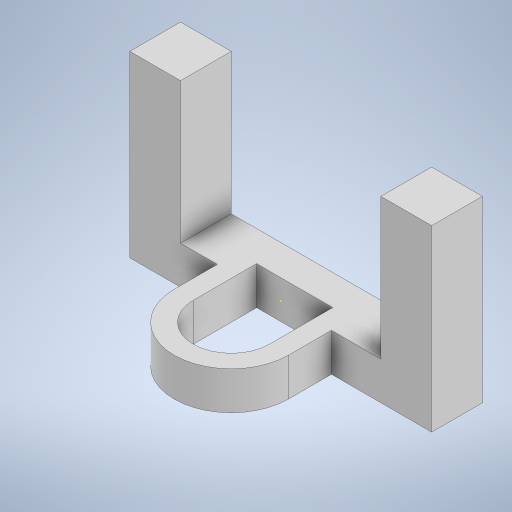
# Autodesk Inventor part: 액추에이터 지지대 3D 프린트
Saved by Autodesk Inventor 2024 (Build 280153000, 153)
## iProperties
Created: 2024-06-08
Part Number: 액추에이터 지지대 3D 프린트
Material: 일반
Document SubType Name: Modeling
Designer: kkamin5
Density: 1 g/cm^3
Appearance: 기본값
Author: kkamin5
Autodesk Inventor part; units mm, degrees
ref_plane "YZ Plane" through (0, 0, 0) normal (1, 0, 0) x (0, 1, 0)
ref_plane "XZ Plane" through (0, 0, 0) normal (0, 1, 0) x (-1, 0, 0)
ref_plane "XY Plane" through (0, 0, 0) normal (0, 0, 1) x (1, 0, 0)
sketch "스케치1" plane through (0, 0, 0) normal (0, 1, 0) x (-1, 0, 0)
  arc A0 (25, 17) -> (-20, 17) centre (2.5, 17) ccw
  arc A1 (17.5, 17) -> (-12.5, 17) centre (2.5, 17) ccw
  line L0 (17.5, 17) -> (-12.5, 17)
  line L1 (-20, 17) -> (-20, 0)
  line L2 (-20, -20) -> (25, -20)
  line L3 (25, 0) -> (25, 17)
  line L4 (-12.5, 17) -> (17.5, 17)
  line L5 (17.5, 17) -> (17.5, 0)
  line L6 (17.5, 0) -> (-12.5, 0)
  line L7 (-12.5, 0) -> (-12.5, 17)
  line L8 (59.5, -20) -> (-59.5, -20)
  line L9 (-59.5, -20) -> (-59.5, 0)
  line L10 (59.5, 0) -> (59.5, -20)
  line L11 (25, 0) -> (59.5, 0)
  line L12 (-59.5, 0) -> (-20, 0)
  line L13 (-12.5, 0) -> (17.5, 0)
  line L14 (17.5, 0) -> (-12.5, 0)
  line L15 (-12.5, 0) -> (-12.5, -8)
  line L16 (-12.5, -8) -> (17.5, -8)
  line L17 (17.5, -8) -> (17.5, 0)
  point P0 (0, 0)
  point P1 (0, 17)
  point P2 (-59.5, -10)
  dimension "d1" = 30
  dimension "d2" = 45
  dimension "d3" = 0
  dimension "d4" = 17
  dimension "d5" = 37
  dimension "d6" = 119
  dimension "d10" = 20
  dimension "d11" = 22.5
  dimension "d12" = 0
  dimension "d13" = 59.5
  dimension "d14" = 8
  dimension "d15" = 39.5
  constraints: 36 end point, 10 parallel, 4 horizontal, 4 perpendicular, 4 point on circle, 3 collinear, 3 tangent, 2 centre point, 2 point on line, 1 coincident, 1 midpoint
  measures "d1" diameter of A1
  measures "d2" distance of L2.start L2.end
  measures "d3" horizontal distance of point (0, 17) point (0, 0)
  measures "d4" distance of L0.start L5.end
  measures "d5" distance of L2.end L3.end
  measures "d6" distance of L8.start L8.end
  measures "d10" distance of L10.start L8.start
  measures "d11" radius of A0
  measures "d12" distance from line of point (0, 0) L6
  measures "d13" distance from line of point (0, 0) L10
  measures "d14" distance of L15.end L14.end
  measures "d15" distance between parallel lines of L9 L1
extrude "돌출1" add sketch "스케치1" along normal blind 15
sketch "스케치2" plane through (0, 15, 0) normal (0, 1, 0) x (1, 0, 0)
  point P0 (0, 0)
sketch "스케치3" plane through (0, 15, 0) normal (0, 1, 0) x (1, 0, 0)
  line L0 (-39.5, 0) -> (-59.5, 0)
  line L1 (-59.5, 0) -> (-59.5, 20)
  line L2 (-59.5, 20) -> (-39.5, 20)
  line L3 (-39.5, 20) -> (-39.5, 0)
  line L4 (-39.5, 0) -> (-59.5, 20) construction
  line L5 (-59.5, 0) -> (-39.5, 20) construction
  line L6 (-59.5, 20) -> (-59.5, 0) projected
  line L7 (-59.5, 0) -> (-25, 0) projected
  line L8 (0, 0) -> (0, 5.3551)
  line L9 (39.5, 0) -> (59.5, 0)
  line L10 (59.5, 0) -> (59.5, 20)
  line L11 (59.5, 20) -> (39.5, 20)
  line L12 (39.5, 20) -> (39.5, 0)
  line L13 (39.5, 0) -> (59.5, 20) construction
  line L14 (59.5, 0) -> (39.5, 20) construction
  line L15 (59.5, 20) -> (59.5, 0)
  line L16 (59.5, 0) -> (25, 0)
  point P0 (-49.5, 10)
  point P1 (-49.5, 0)
  point P2 (49.5, 10)
  point P3 (49.5, 0)
  dimension "d16" = 20
  dimension "d17" = 20
  dimension "d18" = 0
  dimension "d19" = 0
  constraints: 30 end point, 9 symmetric about line, 3 midpoint, 2 parallel, 1 horizontal, 1 perpendicular, 1 vertical
  measures "d16" distance of L1.end L2.end
  measures "d17" distance of L0.end L1.end
  measures "d18" distance between parallel lines of L6 L1
  measures "d19" distance from line of L7 point (-49.5, 0)
extrude "돌출2" add sketch "스케치3" along normal blind 55.5
equation "\"d13\" = 0.5 * d6"
